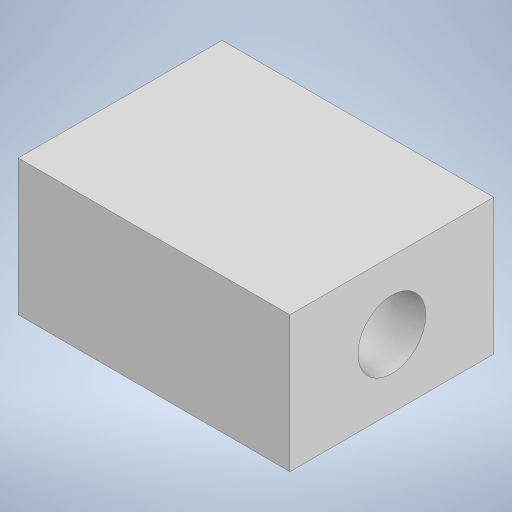
# Autodesk Inventor part: stop_block
Saved by Autodesk Inventor 2024.3 (Build 283343000, 343)
## iProperties
Created: 2024-08-04
Part Number: stop_block
Material: Generic
Document SubType Name: Modeling
Designer: compu
Density: 1 g/cm^3
Appearance: Default
Author: compu
Autodesk Inventor part; units mm, degrees
ref_plane "YZ Plane" through (0, 0, 0) normal (1, 0, 0) x (0, 1, 0)
ref_plane "XZ Plane" through (0, 0, 0) normal (0, 1, 0) x (-1, 0, 0)
ref_plane "XY Plane" through (0, 0, 0) normal (0, 0, 1) x (1, 0, 0)
sketch "Sketch1" plane through (0, 0, 0) normal (0, 1, 0) x (-1, 0, 0)
  line L0 (10, -7.5) -> (-10, -7.5)
  line L1 (-10, -7.5) -> (-10, 7.5)
  line L2 (-10, 7.5) -> (10, 7.5)
  line L3 (10, 7.5) -> (10, -7.5)
  line L4 (14, 0) -> (-14, 0) projected
  line L5 (0, -10.5) -> (0, 10.5) projected
  point P0 (0, 0)
  dimension "d0" = 15
  dimension "d1" = 20
  constraints: 8 end point, 2 parallel, 1 horizontal, 1 perpendicular, 2 other
  measures "d0" distance of L0.end L1.end
  measures "d1" distance of L0.start L0.end
extrude "Extrusion1" add sketch "Sketch1" along normal blind 10
sketch "Sketch2" plane through (10, 0, 7.5) normal (1, 0, 0) x (0, 0, -1)
  line L0 (0, 0) -> (15, 0) projected
  line L1 (15, 0) -> (15, 10) projected
  line L2 (0, 10) -> (15, 10) projected
  line L3 (0, 0) -> (0, 10) projected
  circle A0 centre (7.5, 5) radius 2.5
  line L4 (15, 10) -> (0, 0) construction
  line L5 (0, 10) -> (15, 0) construction
  point P0 (7.5, 0)
  dimension "d4" = 5
  constraints: 4 end point, 3 midpoint, 1 centre point, 1 coincident
  measures "d4" diameter of A0
extrude "Extrusion2" cut sketch "Sketch2" against normal through all contours A0
body "Solid1"
